Autodesk Fusion 360 part; units mm, degrees
(part 4 of 4)
  constraint coincident L729.end L734
  constraint perpendicular L729 L734
  constraint perpendicular L626 L768
  constraint coincident L630.end L658
  constraint perpendicular L630 L658
  constraint equal L626 L630
  constraint equal L626 L683
  constraint equal L626 L729
  constraint tangent L658 A42
  constraint tangent L690 A42
  constraint tangent A42 L768
  constraint coincident L694.end A42
  constraint coincident L694.start A42
  constraint coincident L622.end A42
  constraint coincident L622.start A42
  constraint tangent A42 L734
  constraint coincident P66 L622
  constraint coincident P66 L694
  constraint coincident P66 P37
  constraint vertical L701
  constraint perpendicular L648 L737
  constraint perpendicular L623 L718
  constraint perpendicular L623 L715
  constraint perpendicular L623 L672
  constraint perpendicular L648 L758
  constraint perpendicular L692 L737
  constraint equal L701 L718
  constraint equal L715 L718
  constraint equal L648 L718
  constraint symmetric L685.start L627.end L623
  constraint symmetric L672.start L627.start L623
  constraint symmetric L665.end L653.start L623
  constraint symmetric L665.start L653.end L623
  constraint symmetric L701.start L677.start L737
  constraint symmetric L677.end L673.start L737
  constraint symmetric L625.end L647.start L737
  constraint equal L672 L692
  constraint equal L692 L758
  constraint parallel L636 L648
  constraint equal L636 L692
  constraint symmetric L625.start L636.start L737
  constraint coincident L673.end L701
  constraint perpendicular L673 L701
  constraint coincident L644.end L718
  constraint coincident L676.end L715
  constraint perpendicular L676 L715
  constraint perpendicular L644 L718
  constraint coincident L650.end L648
  constraint perpendicular L648 L650
  constraint equal L644 L650
  constraint equal L644 L673
  constraint equal L644 L676
  constraint tangent L648 A43
  constraint tangent L701 A43
  constraint tangent L718 A43
  constraint coincident L737.end A43
  constraint coincident L737.start A43
  constraint coincident L623.end A43
  constraint coincident L623.start A43
  constraint tangent L715 A43
  constraint coincident P65 L623
  constraint coincident P65 L737
  constraint coincident P65 P38
  constraint vertical L649
  constraint perpendicular L643 L671
  constraint perpendicular L689 L691
  constraint perpendicular L678 L691
  constraint perpendicular L691 L725
  constraint perpendicular L643 L763
  constraint perpendicular L661 L671
  constraint equal L649 L689
  constraint equal L678 L689
  constraint equal L643 L689
  constraint symmetric L689.end L628.start L691
  constraint symmetric L640.start L628.end L691
  constraint symmetric L678.end L678.start L691
  constraint symmetric L698.start L704.end L691
  constraint symmetric L649.start L649.end L671
  constraint symmetric L661.start L645.start L671
  constraint symmetric L643.end L643.start L671
  constraint equal L661 L725
  constraint equal L661 L763
  constraint parallel L643 L724
  constraint equal L661 L724
  constraint symmetric L699.start L724.start L671
  constraint coincident L645.end L649
  constraint perpendicular L645 L649
  constraint coincident L640.end L689
  constraint coincident L705.end L678
  constraint perpendicular L678 L705
  constraint perpendicular L640 L689
  constraint coincident L720.end L643
  constraint perpendicular L643 L720
  constraint equal L640 L720
  constraint equal L640 L645
  constraint equal L640 L705
  constraint tangent A38 L643
  constraint tangent A38 L649
  constraint tangent A38 L689
  constraint coincident L671.end A38
  constraint coincident L671.start A38
  constraint coincident L691.end A38
  constraint coincident L691.start A38
  constraint tangent A38 L678
  constraint coincident P64 L691
  constraint coincident P64 L671
  constraint coincident P64 P39
  constraint vertical L660
  constraint perpendicular L687 L706
  constraint perpendicular L659 L756
  constraint perpendicular L659 L713
  constraint perpendicular L659 L761
  constraint perpendicular L651 L706
  constraint perpendicular L687 L711
  constraint equal L660 L756
  constraint equal L713 L756
  constraint equal L706 L756
  constraint symmetric L664.start L666.end L659
  constraint symmetric L664.end L632.start L659
  constraint symmetric L621.end L629.start L659
  constraint symmetric L621.start L629.end L659
  constraint symmetric L660.start L660.end L687
  constraint symmetric L711.start L668.start L687
  constraint symmetric L684.end L637.start L687
  constraint equal L711 L761
  constraint equal L651 L711
  constraint parallel L706 L714
  constraint equal L711 L714
  constraint symmetric L637.end L646.start L687
  constraint coincident L668.end L660
  constraint perpendicular L660 L668
  constraint coincident L632.end L756
  constraint coincident L669.end L713
  constraint perpendicular L669 L713
  constraint perpendicular L632 L756
  constraint coincident L646.end L706
  constraint perpendicular L646 L706
  constraint equal L632 L646
  constraint equal L632 L668
  constraint equal L632 L669
  constraint tangent A39 L706
  constraint tangent L660 A39
  constraint tangent A39 L756
  constraint coincident L687.end A39
  constraint coincident L687.start A39
  constraint coincident L659.end A39
  constraint coincident L659.start A39
  constraint tangent A39 L713
  constraint coincident P63 L659
  constraint coincident P63 L687
  constraint coincident P63 P36
  constraint vertical L693
  constraint perpendicular L657 L785
  constraint perpendicular L654 L777
  constraint perpendicular L654 L784
  constraint perpendicular L654 L782
  constraint perpendicular L657 L781
  constraint perpendicular L712 L785
  constraint equal L693 L777
  constraint equal L777 L784
  constraint equal L657 L777
  constraint symmetric L655.end L710.start L654
  constraint symmetric L710.end L655.start L654
  constraint symmetric L784.end L749.end L654
  constraint symmetric L781.start L736.start L654
  constraint symmetric L693.start L693.end L785
  constraint symmetric L712.end L712.start L785
  constraint symmetric L635.end L657.start L785
  constraint equal L712 L782
  constraint equal L712 L781
  constraint parallel L634 L657
  constraint equal L634 L712
  constraint symmetric L634.start L634.end L785
  constraint coincident L747.end L693
  constraint perpendicular L693 L747
  constraint coincident L792.end L777
  constraint coincident L736.end L784
  constraint perpendicular L736 L784
  constraint perpendicular L777 L792
  constraint coincident L776.end L657
  constraint perpendicular L657 L776
  constraint equal L776 L792
  constraint equal L747 L792
  constraint equal L736 L792
  constraint tangent L657 A45
  constraint tangent L693 A45
  constraint tangent L777 A45
  constraint coincident L785.end A45
  constraint coincident L785.start A45
  constraint coincident L654.end A45
  constraint coincident L654.start A45
  constraint tangent L784 A45
  constraint coincident P62 L654
  constraint coincident P62 L785
  constraint coincident P62 P40
  constraint vertical L778
  constraint perpendicular L641 L735
  constraint perpendicular L780 L787
  constraint perpendicular L787 L793
  constraint perpendicular L620 L787
  constraint perpendicular L641 L789
  constraint perpendicular L735 L783
  constraint equal L778 L780
  constraint equal L780 L793
  constraint equal L641 L780
  constraint symmetric L656.end L780.start L787
  constraint symmetric L620.start L620.end L787
  constraint symmetric L788.end L642.start L787
  constraint symmetric L775.start L642.end L787
  constraint symmetric L624.end L774.start L735
  constraint symmetric L624.start L774.end L735
  constraint symmetric L641.end L641.start L735
  constraint equal L620 L783
  constraint equal L783 L789
  constraint parallel L641 L779
  constraint equal L779 L783
  constraint symmetric L697.start L722.end L735
  constraint coincident L791.end L778
  constraint perpendicular L778 L791
  constraint coincident L795.end L780
  constraint coincident L775.end L793
  constraint perpendicular L775 L793
  constraint perpendicular L780 L795
  constraint coincident L731.end L641
  constraint perpendicular L641 L731
  constraint equal L731 L795
  constraint equal L791 L795
  constraint equal L775 L795
  constraint tangent L641 A44
  constraint tangent A44 L778
  constraint tangent A44 L780
  constraint coincident L735.end A44
  constraint coincident L735.start A44
  constraint coincident L787.end A44
  constraint coincident L787.start A44
  constraint tangent A44 L793
  constraint coincident P61 L787
  constraint coincident P61 L735
  constraint coincident P61 P41
  constraint vertical L723
  constraint perpendicular L638 L679
  constraint perpendicular L633 L695
  constraint perpendicular L633 L748
  constraint perpendicular L633 L702
  constraint perpendicular L638 L674
  constraint perpendicular L667 L679
  constraint equal L695 L723
  constraint equal L695 L748
  constraint equal L638 L695
  constraint symmetric L682.end L631.start L633
  constraint symmetric L662.start L631.end L633
  constraint symmetric L726.start L700.end L633
  constraint symmetric L674.end L674.start L633
  constraint symmetric L723.start L723.end L679
  constraint symmetric L667.start L667.end L679
  constraint symmetric L638.end L638.start L679
  constraint equal L667 L702
  constraint equal L667 L674
  constraint parallel L638 L738
  constraint equal L667 L738
  constraint symmetric L733.start L728.end L679
  constraint coincident L750.end L723
  constraint perpendicular L723 L750
  constraint coincident L662.end L695
  constraint coincident L686.end L748
  constraint perpendicular L686 L748
  constraint perpendicular L662 L695
  constraint coincident L757.end L638
  constraint perpendicular L638 L757
  constraint equal L662 L757
  constraint equal L662 L750
  constraint equal L662 L686
  constraint tangent L638 A40
  constraint tangent A40 L723
  constraint tangent L695 A40
  constraint coincident L679.end A40
  constraint coincident L679.start A40
  constraint coincident L633.end A40
  constraint coincident L633.start A40
  constraint tangent A40 L748
  constraint coincident P60 L633
  constraint coincident P60 L679
  constraint coincident P60 P42
  constraint vertical L760
  constraint perpendicular L764 L772
  constraint perpendicular L745 L770
  constraint perpendicular L770 L773
  constraint perpendicular L767 L770
  constraint perpendicular L766 L772
  constraint perpendicular L739 L764
  constraint equal L745 L760
  constraint equal L745 L773
  constraint equal L745 L772
  constraint symmetric L719.start L703.end L770
  constraint symmetric L719.end L703.start L770
  constraint symmetric L752.end L721.start L770
  constraint symmetric L721.end L752.start L770
  constraint symmetric L760.end L716.end L764
  constraint symmetric L739.start L716.start L764
  constraint symmetric L753.end L754.start L764
  constraint equal L739 L767
  constraint equal L739 L766
  constraint parallel L744 L772
  constraint equal L739 L744
  constraint symmetric L727.start L744.start L764
  constraint coincident L765.end L760
  constraint perpendicular L760 L765
  constraint coincident L742.end L745
  constraint coincident L769.end L773
  constraint perpendicular L769 L773
  constraint perpendicular L742 L745
  constraint coincident L727.end L772
  constraint perpendicular L727 L772
  constraint equal L727 L742
  constraint equal L742 L765
  constraint equal L742 L769
  constraint tangent A41 L772
  constraint tangent A41 L760
  constraint tangent A41 L745
  constraint coincident L764.end A41
  constraint coincident L764.start A41
  constraint coincident L770.end A41
  constraint coincident L770.start A41
  constraint tangent A41 L773
  constraint coincident P59 L770
  constraint coincident P59 L764
  constraint coincident P59 P43
  constraint vertical L811
  constraint perpendicular L818 L873
  constraint perpendicular L860 L879
  constraint perpendicular L834 L879
  constraint perpendicular L817 L879
  constraint perpendicular L854 L873
  constraint perpendicular L818 L832
  constraint equal L811 L860
  constraint equal L834 L860
  constraint equal L860 L873
  constraint symmetric L860.end L824.start L879
  constraint symmetric L817.end L817.start L879
  constraint symmetric L834.end L816.end L879
  constraint symmetric L796.start L854.start L879
  constraint symmetric L811.start L811.end L818
  constraint symmetric L812.end L821.start L818
  constraint symmetric L823.end L873.start L818
  constraint equal L817 L832
  constraint equal L832 L854
  constraint parallel L872 L873
  constraint equal L832 L872
  constraint symmetric L823.start L872.start L818
  constraint coincident L829.end L811
  constraint perpendicular L811 L829
  constraint coincident L870.end L860
  constraint coincident L796.end L834
  constraint perpendicular L796 L834
  constraint perpendicular L860 L870
  constraint coincident L867.end L873
  constraint perpendicular L867 L873
  constraint equal L867 L870
  constraint equal L829 L870
  constraint equal L796 L870
  constraint tangent A49 L873
  constraint tangent L811 A49
  constraint tangent A49 L860
  constraint coincident L818.end A49
  constraint coincident L818.start A49
  constraint coincident L879.end A49
  constraint coincident L879.start A49
  constraint tangent L834 A49
  constraint coincident P67 L879
  constraint coincident P67 L818
  constraint coincident P67 P46
  constraint vertical L826
  constraint perpendicular L842 L853
  constraint perpendicular L820 L825
  constraint perpendicular L825 L833
  constraint perpendicular L825 L845
  constraint perpendicular L806 L853
  constraint perpendicular L842 L863
  constraint equal L820 L826
  constraint equal L820 L833
  constraint equal L820 L853
  constraint symmetric L820.start L798.end L825
  constraint symmetric L845.start L798.start L825
  constraint symmetric L805.end L804.start L825
  constraint symmetric L804.end L805.start L825
  constraint symmetric L826.end L819.end L842
  constraint symmetric L835.end L797.start L842
  constraint symmetric L840.end L813.start L842
  constraint equal L845 L863
  constraint equal L806 L863
  constraint parallel L853 L866
  constraint equal L863 L866
  constraint symmetric L840.start L813.end L842
  constraint coincident L797.end L826
  constraint perpendicular L797 L826
  constraint coincident L852.end L820
  constraint coincident L814.end L833
  constraint perpendicular L814 L833
  constraint perpendicular L820 L852
  constraint coincident L846.end L853
  constraint perpendicular L846 L853
  constraint equal L846 L852
  constraint equal L797 L852
  constraint equal L814 L852
  constraint tangent A47 L853
  constraint tangent L826 A47
  constraint tangent L820 A47
  constraint coincident L842.end A47
  constraint coincident L842.start A47
  constraint coincident L825.end A47
  constraint coincident L825.start A47
  constraint tangent A47 L833
  constraint coincident P56 L825
  constraint coincident P56 L842
  constraint coincident P56 P47
  constraint vertical L800
  constraint perpendicular L822 L874
  constraint perpendicular L830 L881
  constraint perpendicular L828 L881
  constraint perpendicular L831 L881
  constraint perpendicular L827 L874
  constraint perpendicular L822 L848
  constraint equal L800 L830
  constraint equal L828 L830
  constraint equal L830 L874
  constraint symmetric L830.start L830.end L881
  constraint symmetric L831.end L831.start L881
  constraint symmetric L828.start L828.end L881
  constraint symmetric L827.start L807.start L881
  constraint symmetric L800.start L800.end L822
  constraint symmetric L847.end L848.end L822
  constraint symmetric L874.start L871.end L822
  constraint equal L831 L848
  constraint equal L827 L848
  constraint parallel L874 L880
  constraint equal L848 L880
  constraint symmetric L869.start L880.start L822
  constraint coincident L851.end L800
  constraint perpendicular L800 L851
  constraint coincident L883.end L830
  constraint coincident L807.end L828
  constraint perpendicular L807 L828
  constraint perpendicular L830 L883
  constraint coincident L869.end L874
  constraint perpendicular L869 L874
  constraint equal L869 L883
  constraint equal L851 L883
  constraint equal L807 L883
  constraint tangent A46 L874
  constraint tangent L800 A46
  constraint tangent A46 L830
  constraint coincident L822.end A46
  constraint coincident L822.start A46
  constraint coincident L881.end A46
  constraint coincident L881.start A46
  constraint tangent A46 L828
  constraint coincident P58 L881
  constraint coincident P58 L822
  constraint coincident P58 P44
  constraint vertical L858
  constraint perpendicular L810 L843
  constraint perpendicular L802 L809
  constraint perpendicular L809 L839
  constraint perpendicular L799 L809
  constraint perpendicular L810 L864
  constraint perpendicular L808 L843
  constraint equal L802 L858
  constraint equal L802 L839
  constraint equal L802 L810
  constraint symmetric L802.end L802.start L809
  constraint symmetric L799.start L799.end L809
  constraint symmetric L839.start L839.end L809
  constraint symmetric L855.start L857.end L809
  constraint symmetric L803.start L850.end L843
  constraint symmetric L808.end L803.end L843
  constraint symmetric L810.end L801.start L843
  constraint equal L799 L808
  constraint equal L808 L864
  constraint parallel L810 L836
  constraint equal L808 L836
  constraint symmetric L801.end L815.start L843
  constraint coincident L841.end L858
  constraint perpendicular L841 L858
  constraint coincident L838.end L802
  constraint coincident L861.end L839
  constraint perpendicular L839 L861
  constraint perpendicular L802 L838
  constraint coincident L849.end L810
  constraint perpendicular L810 L849
  constraint equal L838 L849
  constraint equal L838 L841
  constraint equal L838 L861
  constraint tangent L810 A48
  constraint tangent A48 L858
  constraint tangent L802 A48
  constraint coincident L843.end A48
  constraint coincident L843.start A48
  constraint coincident L809.end A48
  constraint coincident L809.start A48
  constraint tangent A48 L839
  constraint coincident P57 L809
  constraint coincident P57 L843
  constraint coincident P57 P45
  constraint equal A42 A50
  constraint equal A43 A51
  constraint equal A38 A52
  constraint equal A39 A53
  constraint equal A45 A54
  constraint equal A44 A55
  constraint equal A40 A56
  constraint equal A41 A57
  constraint equal A46 A58
  constraint equal A48 A59
  constraint equal A47 A60
  constraint equal A49 A61
  constraint equal A37 A62
  constraint equal A34 A63
  constraint equal A35 A64
  constraint equal A36 A65
  constraint equal A33 A66
  constraint equal A32 A67
  constraint equal A31 A68
  constraint equal A30 A69
  measures "d105" distance of L8.start L8.end
  measures "d106" distance of L10.end L11.end
  measures "d371" distance of L11.end L23.end
  measures "d372" distance of L37.start L36.end
  measures "d373" distance of L37.end L32.start
  measures "d374" distance of L32.end L32.start
  measures "d375" distance of L51.start L48.end
  measures "d376" distance of L48.start L51.end
  measures "d377" distance of L48.start L63.end
  measures "d378" distance of L73.start L70.end
  measures "d379" distance of L70.start L73.end
  measures "d380" distance of L70.start L85.end
  measures "d381" distance of L95.start L92.end
  measures "d382" distance of L92.start L95.end
  measures "d383" distance of L92.start L107.end
  measures "d384" distance of L117.start L114.end
  measures "d385" distance of L114.start L117.end
  measures "d386" distance of L114.start L129.end
  measures "d387" distance of L139.start L136.end
  measures "d388" distance of L136.start L139.end
  measures "d389" distance of L136.start L151.end
  measures "d390" distance of L161.start L158.end
  measures "d391" distance of L158.start L161.end
  measures "d392" distance of L158.start L173.end
  measures "d393" distance of L183.start L180.end
  measures "d394" distance of L180.start L183.end
  measures "d395" distance of L180.start L195.end
  measures "d396" distance of L205.start L202.end
  measures "d397" distance of L202.start L205.end
  measures "d398" distance of L202.start L217.end
  measures "d504" distance of L224.start L235.end
  measures "d505" distance of L230.start L224.end
  measures "d506" distance of L230.start L230.end
  measures "d507" distance of L246.start L257.end
  measures "d508" distance of L252.start L246.end
  measures "d509" distance of L252.start L252.end
  measures "d510" distance of L268.start L279.end
  measures "d511" distance of L274.start L268.end
  measures "d512" distance of L274.start L274.end
  measures "d513" distance of L290.start L301.end
  measures "d514" distance of L296.start L290.end
  measures "d515" distance of L296.start L296.end
  measures "d516" distance of L312.start L323.end
  measures "d517" distance of L318.start L312.end
  measures "d518" distance of L318.start L318.end
  measures "d519" distance of L334.start L345.end
  measures "d520" distance of L340.start L334.end
  measures "d521" distance of L340.start L340.end
  measures "d522" distance of L356.start L367.end
  measures "d523" distance of L362.start L356.end
  measures "d524" distance of L362.start L362.end
  measures "d525" distance of L378.start L389.end
  measures "d526" distance of L384.start L378.end
  measures "d527" distance of L384.start L384.end
  measures "d528" distance of L400.start L411.end
  measures "d529" distance of L406.start L400.end
  measures "d530" distance of L406.start L406.end
  measures "d531" distance of L422.start L433.end
  measures "d532" distance of L428.start L422.end
  measures "d533" distance of L428.start L428.end
  measures "d568" distance of L450.end L452.start
  measures "d569" distance of L450.start L459.end
  measures "d570" distance of L450.start L457.end
  measures "d571" distance of L477.end L481.start
  measures "d572" distance of L477.start L482.start
  measures "d573" distance of L477.start L478.end
  measures "d574" distance of L495.end L499.start
  measures "d575" distance of L495.start L510.start
  measures "d576" distance of L495.start L528.end
  measures "d577" distance of L513.start L513.end
  measures "d578" distance of L496.start L496.end
  measures "d579" distance of L496.end L523.end
  measures "d580" distance of L542.end L581.start
  measures "d581" distance of L542.start L588.start
  measures "d582" distance of L542.start L561.end
  measures "d583" distance of L576.start L539.end
  measures "d584" distance of L601.end L539.start
  measures "d585" distance of L539.start L540.end
  measures "d586" distance of L549.end L549.start
  measures "d587" distance of L555.start L562.start
  measures "d588" distance of L555.start L555.end
  measures "d589" distance of L591.start L586.end
  measures "d590" distance of L589.start L586.start
  measures "d591" distance of L615.end L586.start
  measures "d592" distance of L652.end L663.start
  measures "d593" distance of L626.start L663.end
  measures "d594" distance of L626.start L626.end
  measures "d595" distance of L685.start L627.end
  measures "d596" distance of L672.start L627.start
  measures "d597" distance of L627.start L644.end
  measures "d598" distance of L689.end L628.start
  measures "d599" distance of L640.start L628.end
  measures "d600" distance of L640.start L640.end
  measures "d601" distance of L664.start L666.end
  measures "d602" distance of L664.end L632.start
  measures "d603" distance of L632.end L632.start
  measures "d604" distance of L655.end L710.start
  measures "d605" distance of L710.end L655.start
  measures "d606" distance of L792.end L655.start
  measures "d607" distance of L656.end L780.start
  measures "d608" distance of L620.start L620.end
  measures "d609" distance of L620.end L795.end
  measures "d610" distance of L682.end L631.start
  measures "d611" distance of L662.start L631.end
  measures "d612" distance of L662.start L662.end
  measures "d613" distance of L719.start L703.end
  measures "d614" distance of L719.end L703.start
  measures "d615" distance of L742.end L703.start
  measures "d616" distance of L860.end L824.start
  measures "d617" distance of L817.end L817.start
  measures "d618" distance of L817.end L870.end
  measures "d619" distance of L820.start L798.end
  measures "d620" distance of L845.start L798.start
  measures "d621" distance of L852.end L798.start
  measures "d622" distance of L830.start L830.end
  measures "d623" distance of L831.end L831.start
  measures "d624" distance of L831.end L883.end
  measures "d625" distance of L802.end L802.start
  measures "d626" distance of L799.start L799.end
  measures "d627" distance of L799.end L838.end
extrude "돌출4" add sketch "스케치1" along normal blind 0.4 contours L0 L1 L2 L3 | L40 L41 L42 L43
extrude "돌출7" add sketch "스케치1" along normal blind 0.4 and the other way blind 0 contours A42 | A43
extrude "돌출6" cut sketch "스케치2" along normal through all contours A40 | L0 L3 L160 | L0 L3 A0 L160 | L0 L1 A0 | A0 | L2 L3 A0 | L1 L2 A0 | A44 | L4 L7 L174 | L4 L7 A1 L174 | L4 L5 A1 | A1 | L6 L7 A1 | L5 L6 A1 | A45 | L8 L11 L175 | L8 L11 A2 L175 | L8 L9 A2 | A2 | L10 L11 A2 | L9 L10 A2 | A46 | L12 L15 L176 | L12 L15 A3 L176 | L12 L13 A3 | A3 | L14 L15 A3 | L13 L14 A3 | A47 | L16 L19 L177 | L16 L19 A4 L177 | L16 L17 A4 | A4 | L18 L19 A4 | L17 L18 A4 | A48 | L20 L23 L178 | L20 L23 A5 L178 | L20 L21 A5 | A5 | L22 L23 A5 | L21 L22 A5 | A49 | L24 L27 L179 | L24 L27 A6 L179 | L24 L25 A6 | A6 | L26 L27 A6 | L25 L26 A6 | A50 | L28 L31 L180 | L28 L31 A7 L180 | L28 L29 A7 | A7 | L30 L31 A7 | L29 L30 A7 | A51 | L32 L35 L181 | L32 L35 A8 L181 | L32 L33 A8 | A8 | L34 L35 A8 | L33 L34 A8 | A52 | L36 L39 L182 | L36 L39 A9 L182 | L36 L37 A9 | A9 | L38 L39 A9 | L37 L38 A9 | A53 | L40 L43 L192 | L40 L43 A10 L192 | L40 L41 A10 | A10 | L42 L43 A10 | L41 L42 A10 | A54 | L44 L47 L169 | L44 L47 A11 L169 | L44 L45 A11 | A11 | L46 L47 A11 | L45 L46 A11 | A55 | L48 L51 L193 | L48 L51 A12 L193 | L48 L49 A12 | A12 | L50 L51 A12 | L49 L50 A12 | A56 | L52 L55 L170 | L52 L55 A13 L170 | L52 L53 A13 | A13 | L54 L55 A13 | L53 L54 A13 | A57 | L56 L59 L194 | L56 L59 A14 L194 | L56 L57 A14 | A14 | L58 L59 A14 | L57 L58 A14 | A58 | L60 L63 L171 | L60 L63 A15 L171 | L60 L61 A15 | A15 | L62 L63 A15 | L61 L62 A15 | A59 | L64 L67 L195 | L64 L67 A16 L195 | L64 L65 A16 | A16 | L66 L67 A16 | L65 L66 A16 | A60 | L68 L71 L172 | L68 L71 A17 L172 | L68 L69 A17 | A17 | L70 L71 A17 | L69 L70 A17 | A61 | L72 L75 L196 | L72 L75 A18 L196 | L72 L73 A18 | A18 | L74 L75 A18 | L73 L74 A18 | A42 | L76 L79 L162 | L76 L79 A19 L162 | L76 L77 A19 | A19 | L78 L79 A19 | L77 L78 A19 | A69 | L80 L83 L213 | L80 L83 A29 L213 | L80 L81 A29 | A29 | L82 L83 A29 | L81 L82 A29 | A70 | L84 L87 L212 | L84 L87 A28 L212 | L84 L85 A28 | A28 | L86 L87 A28 | L85 L86 A28 | A67 | L88 L91 L211 | L88 L91 A27 L211 | L88 L89 A27 | A27 | L90 L91 A27 | L89 L90 A27 | A68 | L92 L95 L210 | L92 L95 A26 L210 | L92 L93 A26 | A26 | L94 L95 A26 | L93 L94 A26 | A65 | L96 L99 L209 | L96 L99 A25 L209 | L96 L97 A25 | A25 | L98 L99 A25 | L97 L98 A25 | A66 | L100 L103 L208 | L100 L103 A23 L208 | L100 L101 A23 | A23 | L102 L103 A23 | L101 L102 A23 | A63 | L104 L107 L207 | L104 L107 A24 L207 | L104 L105 A24 | A24 | L106 L107 A24 | L105 L106 A24 | A64 | L108 L111 L173 | L108 L111 A22 L173 | L108 L109 A22 | A22 | L110 L111 A22 | L109 L110 A22 | A62 | L112 L115 L206 | L112 L115 A21 L206 | L112 L113 A21 | A21 | L114 L115 A21 | L113 L114 A21 | A41 | L116 L119 L165 | L116 L119 A20 L165 | L116 L117 A20 | A20 | L118 L119 A20 | L117 L118 A20 | A79 | L120 L123 L231 | L120 L123 A30 L231 | L120 L121 A30 | A30 | L122 L123 A30 | L121 L122 A30 | A78 | L124 L127 L230 | L124 L127 A31 L230 | L124 L125 A31 | A31 | L126 L127 A31 | L125 L126 A31 | A77 | L128 L131 L229 | L128 L131 A32 L229 | L128 L129 A32 | A32 | L130 L131 A32 | L129 L130 A32 | A76 | L132 L135 L228 | L132 L135 A33 L228 | L132 L133 A33 | A33 | L134 L135 A33 | L133 L134 A33 | A75 | L136 L139 L227 | L136 L139 A34 L227 | L136 L137 A34 | A34 | L138 L139 A34 | L137 L138 A34 | A74 | L140 L143 L226 | L140 L143 A35 L226 | L140 L141 A35 | A35 | L142 L143 A35 | L141 L142 A35 | A73 | L144 L147 L225 | L144 L147 A36 L225 | L144 L145 A36 | A36 | L146 L147 A36 | L145 L146 A36 | A72 | L148 L151 L224 | L148 L151 A37 L224 | L148 L149 A37 | A37 | L150 L151 A37 | L149 L150 A37 | A71 | L152 L155 L223 | L152 L155 A38 L223 | L152 L153 A38 | A38 | L154 L155 A38 | L153 L154 A38 | A43 | L156 L159 L167 | L156 L159 A39 L167 | L156 L157 A39 | A39 | L158 L159 A39 | L157 L158 A39
extrude "돌출8" add sketch "스케치2" along normal blind 0.4 contours A40 | L0 L3 L160 | A44 | L4 L7 L174 | A45 | L8 L11 L175 | A46 | L12 L15 L176 | A47 | L16 L19 L177 | A48 | L20 L23 L178 | A49 | L24 L27 L179 | A50 | L28 L31 L180 | A51 | L32 L35 L181 | A52 | L36 L39 L182 | A53 | L40 L43 L192 | A54 | L44 L47 L169 | A55 | L48 L51 L193 | A56 | L52 L55 L170 | A57 | L56 L59 L194 | A58 | L60 L63 L171 | A59 | L64 L67 L195 | A60 | L68 L71 L172 | A61 | L72 L75 L196 | A42 | L76 L79 L162 | A69 | L80 L83 L213 | A70 | L84 L87 L212 | A67 | L88 L91 L211 | A68 | L92 L95 L210 | A65 | L96 L99 L209 | A66 | L100 L103 L208 | A63 | L104 L107 L207 | A64 | L108 L111 L173 | A62 | L112 L115 L206 | A41 | L116 L119 L165 | A79 | L120 L123 L231 | A78 | L124 L127 L230 | A77 | L128 L131 L229 | A76 | L132 L135 L228 | A75 | L136 L139 L227 | A74 | L140 L143 L226 | A73 | L144 L147 L225 | A72 | L148 L151 L224 | A71 | L152 L155 L223 | A43 | L156 L159 L167
extrude "돌출9" add sketch "스케치2" against normal blind 2 contours A40 | A44 | A45 | A46 | A47 | A48 | A49 | A50 | A51 | A52 | A53 | A54 | A55 | A56 | A57 | A58 | A59 | A60 | A61 | A42 | A69 | A70 | A67 | A68 | A65 | A66 | A63 | A64 | A62 | A41 | A79 | A78 | A77 | A76 | A75 | A74 | A73 | A72 | A71 | A43
extrude "돌출11" add sketch "스케치3" along normal blind 0.4 contours L0 L10 L11 L12 | L3 L16 L17 L18 | L1 L19 L20 L21 | L2 L13 L14 L15 | L26 L27 L31 L45 | L28 L34 L40 L44 | L30 L33 L35 L39 | L36 L37 L43 L47 | L48 L51 L52 L56 | L50 L54 L57 L58 | L55 L59 L60 L61 | L66 L67 L68 L69 | L70 L73 L74 L78 | L72 L76 L79 L80 | L77 L81 L82 L83 | L88 L89 L90 L91 | L92 L95 L96 L100 | L94 L98 L101 L102 | L99 L103 L104 L105 | L110 L111 L112 L113 | L114 L117 L118 L122 | L116 L120 L123 L124 | L121 L125 L126 L127 | L132 L133 L134 L135 | L136 L139 L140 L144 | L138 L142 L145 L146 | L143 L147 L148 L149 | L154 L155 L156 L157 | L158 L161 L162 L166 | L160 L164 L167 L168 | L165 L169 L170 L171 | L176 L177 L178 L179 | L180 L183 L184 L188 | L182 L186 L189 L190 | L187 L191 L192 L193 | L198 L199 L200 L201 | L202 L205 L206 L210 | L204 L208 L211 L212 | L209 L213 L214 L215 | L220 L221 L222 L223 | L224 L235 A21 | L224 L242 L243 A21 | L235 L242 A21 | L227 L244 A21 | L229 L231 L244 A21 | L227 L231 A21 | L226 L239 L240 A21 | L234 L240 A21 | L234 L239 A21 | L237 L241 A21 | L228 L232 L237 A21 | L232 L241 A21 | L246 L257 A22 | L246 L264 L265 A22 | L257 L264 A22 | L249 L266 A22 | L251 L253 L266 A22 | L249 L253 A22 | L248 L261 L262 A22 | L256 L262 A22 | L256 L261 A22 | L259 L263 A22 | L250 L254 L259 A22 | L254 L263 A22 | L268 L279 A23 | L268 L286 L287 A23 | L279 L286 A23 | L271 L288 A23 | L273 L275 L288 A23 | L271 L275 A23 | L270 L283 L284 A23 | L278 L284 A23 | L278 L283 A23 | L281 L285 A23 | L272 L276 L281 A23 | L276 L285 A23 | L290 L301 A24 | L290 L308 L309 A24 | L301 L308 A24 | L293 L310 A24 | L295 L297 L310 A24 | L293 L297 A24 | L292 L305 L306 A24 | L300 L306 A24 | L300 L305 A24 | L303 L307 A24 | L294 L298 L303 A24 | L298 L307 A24 | L312 L323 A20 | L312 L330 L331 A20 | L323 L330 A20 | L315 L332 A20 | L317 L319 L332 A20 | L315 L319 A20 | L314 L327 L328 A20 | L322 L328 A20 | L322 L327 A20 | L325 L329 A20 | L316 L320 L325 A20 | L320 L329 A20 | L334 L345 A25 | L334 L352 L353 A25 | L345 L352 A25 | L337 L354 A25 | L339 L341 L354 A25 | L337 L341 A25 | L336 L349 L350 A25 | L344 L350 A25 | L344 L349 A25 | L347 L351 A25 | L338 L342 L347 A25 | L342 L351 A25 | L356 L367 A26 | L356 L374 L375 A26 | L367 L374 A26 | L359 L376 A26 | L361 L363 L376 A26 | L359 L363 A26 | L358 L371 L372 A26 | L366 L372 A26 | L366 L371 A26 | L369 L373 A26 | L360 L364 L369 A26 | L364 L373 A26 | L378 L389 A27 | L378 L396 L397 A27 | L389 L396 A27 | L381 L398 A27 | L383 L385 L398 A27 | L381 L385 A27 | L380 L393 L394 A27 | L388 L394 A27 | L388 L393 A27 | L391 L395 A27 | L382 L386 L391 A27 | L386 L395 A27 | L400 L411 A28 | L400 L418 L419 A28 | L411 L418 A28 | L403 L420 A28 | L405 L407 L420 A28 | L403 L407 A28 | L402 L415 L416 A28 | L410 L416 A28 | L410 L415 A28 | L413 L417 A28 | L404 L408 L413 A28 | L408 L417 A28 | L422 L433 A29 | L422 L440 L441 A29 | L433 L440 A29 | L425 L442 A29 | L427 L429 L442 A29 | L425 L429 A29 | L424 L437 L438 A29 | L432 L438 A29 | L432 L437 A29 | L435 L439 A29 | L426 L430 L435 A29 | L430 L439 A29 | L444 L447 L456 A69 | L444 L453 A69 | L460 L461 L465 A69 | L461 L464 A69 | L447 L453 A69 | L460 L464 A69 | L448 L455 A69 | L449 L451 L455 A69 | L448 L449 A69 | L450 L459 L462 A69 | L452 L459 A69 | L450 L452 A69 | L466 L476 L480 A68 | L466 L470 A68 | L469 L475 L486 A68 | L469 L474 A68 | L470 L476 A68 | L474 L486 A68 | L471 L472 A68 | L471 L473 L487 A68 | L472 L473 A68 | L477 L482 L484 A68 | L481 L484 A68 | L477 L481 A68 | L488 L491 A67 | L491 L493 L529 A67 | L488 L529 A67 | L495 L499 A67 | L495 L510 L518 A67 | L497 L503 L512 A67 | L492 L497 A67 | L499 L518 A67 | L492 L512 A67 | L506 L522 A67 | L505 L506 L508 A67 | L508 L522 A67 | L494 L507 L515 A66 | L494 L501 A66 | L500 L502 L509 A66 | L509 L517 A66 | L501 L515 A66 | L500 L517 A66 | L511 L524 A66 | L511 L516 L525 A66 | L516 L524 A66 | L496 L527 L531 A66 | L513 L527 A66 | L513 L531 A66 | L532 L614 A64 | L570 L587 L614 A64 | L532 L587 A64 | L539 L576 A64 | L539 L601 L609 A64 | L547 L550 L566 A64 | L550 L571 A64 | L576 L601 A64 | L547 L571 A64 | L538 L602 A64 | L538 L556 L567 A64 | L556 L602 A64 | L533 L545 L560 A65 | L533 L535 A65 | L548 L594 L604 A65 | L548 L554 A65 | L535 L545 A65 | L554 L604 A65 | L542 L581 A65 | L542 L588 L592 A65 | L581 L592 A65 | L569 L575 L598 A65 | L574 L575 A65 | L569 L574 A65 | L537 L590 A63 | L537 L544 L563 A63 | L563 L590 A63 | L546 L595 A63 | L568 L585 L595 A63 | L546 L568 A63 | L541 L543 L579 A63 | L543 L564 A63 | L541 L564 A63 | L549 L603 A63 | L562 L596 L603 A63 | L549 L596 A63 | L565 L584 L619 A62 | L565 L616 A62 | L586 L589 L591 A62 | L591 L611 A62 | L584 L616 A62 | L586 L611 A62 | L610 L617 A62 | L608 L613 L617 A62 | L610 L613 A62 | L577 L593 L606 A62 | L577 L605 A62 | L605 L606 A62 | L620 L656 L794 A55 | L780 L794 A55 | L656 L780 A55 | L624 L778 A55 | L624 L774 L783 A55 | L697 L722 L779 A55 | L641 L722 A55 | L774 L778 A55 | L641 L697 A55 | L788 L793 A55 | L642 L788 L789 A55 | L642 L793 A55 | L621 L629 L651 A53 | L621 L713 A53 | L680 L711 L743 A53 | L660 L743 A53 | L629 L713 A53 | L660 L680 A53 | L684 L706 A53 | L637 L684 L714 A53 | L637 L706 A53 | L664 L666 L761 A53 | L664 L756 A53 | L666 L756 A53 | L625 L636 L647 A51 | L625 L648 A51 | L653 L665 L758 A51 | L653 L715 A51 | L647 L648 A51 | L665 L715 A51 | L627 L718 A51 | L627 L672 L685 A51 | L685 L718 A51 | L677 L692 L707 A51 | L677 L701 A51 | L701 L707 A51 | L628 L689 A52 | L628 L725 L741 A52 | L689 L741 A52 | L649 L746 A52 | L661 L670 L746 A52 | L649 L670 A52 | L699 L724 L751 A52 | L643 L751 A52 | L643 L699 A52 | L678 L698 A52 | L698 L704 L763 A52 | L678 L704 A52 | L631 L695 A56 | L631 L682 L702 A56 | L682 L695 A56 | L723 L755 A56 | L667 L740 L755 A56 | L723 L740 A56 | L728 L733 L738 A56 | L638 L728 A56 | L638 L733 A56 | L700 L748 A56 | L674 L700 L726 A56 | L726 L748 A56 | L634 L635 L790 A54 | L657 L790 A54 | L635 L657 A54 | L655 L777 A54 | L655 L710 L782 A54 | L749 L781 L786 A54 | L784 L786 A54 | L710 L777 A54 | L749 L784 A54 | L693 L759 A54 | L712 L730 L759 A54 | L693 L730 A54 | L639 L675 L681 A50 | L639 L658 A50 | L688 L696 L708 A50 | L708 L734 A50 | L658 L675 A50 | L688 L734 A50 | L652 L768 A50 | L652 L663 L732 A50 | L663 L768 A50 | L709 L717 L762 A50 | L690 L762 A50 | L690 L717 A50 | L703 L719 L767 A57 | L703 L745 A57 | L744 L753 L754 A57 | L754 L772 A57 | L719 L745 A57 | L753 L772 A57 | L716 L760 A57 | L716 L739 L771 A57 | L760 L771 A57 | L721 L752 L766 A57 | L721 L773 A57 | L752 L773 A57 | L798 L845 L862 A60 | L798 L820 A60 | L813 L840 L866 A60 | L813 L853 A60 | L820 L862 A60 | L840 L853 A60 | L819 L826 A60 | L819 L835 L863 A60 | L826 L835 A60 | L804 L805 L806 A60 | L804 L833 A60 | L805 L833 A60 | L799 L837 L859 A59 | L802 L837 A59 | L802 L859 A59 | L850 L858 A59 | L803 L808 L850 A59 | L801 L815 L836 A59 | L801 L810 A59 | L803 L858 A59 | L810 L815 A59 | L839 L855 A59 | L855 L857 L864 A59 | L839 L857 A59 | L800 L856 A58 | L800 L847 A58 | L847 L848 L856 A58 | L831 L844 L878 A58 | L830 L844 A58 | L828 L865 A58 | L827 L865 L875 A58 | L830 L878 A58 | L828 L875 A58 | L871 L880 L882 A58 | L874 L882 A58 | L871 L874 A58 | L811 L821 A61 | L811 L812 A61 | L812 L821 L832 A61 | L817 L824 L868 A61 | L824 L860 A61 | L816 L834 A61 | L816 L854 L877 A61 | L860 L868 A61 | L834 L877 A61 | L823 L872 L876 A61 | L873 L876 A61 | L823 L873 A61
move_body "이동1" bodies 1 to x (1, 0, 0) y (0, -1, 0) z (0, 0, -1) at (0, 138, 0.8)
move_body "이동2" bodies 1 to x (1, 0, 0) y (0, 1, 0) z (0, 0, 1) at (0, -69, -0.4)
equation "d6 = RADIUS"
equation "d38 = HEIGHT"
equation "d46 = HEIGHT"
equation "d51 = DEGR"
equation "d55 = DEGR"
equation "d57 = HEIGHT"
equation "d59 = -( COL + 1 mm )"
equation "RADIUS = 10.1 mm"
equation "d63 = DEGR"
equation "d64 = DEGR"
equation "d65 = DEGR"
equation "d66 = DEGR"
equation "d67 = DEGR"
equation "d68 = DEGR"
equation "d69 = DEGR"
equation "d70 = DEGR"
equation "d72 = DEGR"
equation "DEGR = 45 deg"
equation "d74 = DEGR"
equation "d75 = DEGR"
equation "d76 = DEGR"
equation "d77 = DEGR"
equation "d78 = DEGR"
equation "d80 = DEGR"
equation "d81 = DEGR"
equation "d82 = DEGR"
equation "d83 = DEGR"
equation "d84 = DEGR"
equation "d85 = DEGR"
equation "d86 = DEGR"
equation "d87 = DEGR"
equation "d88 = DEGR"
equation "d89 = DEGR"
equation "d91 = DEGR"
equation "d92 = DEGR"
equation "d93 = DEGR"
equation "d94 = DEGR"
equation "d95 = DEGR"
equation "d96 = DEGR"
equation "d97 = DEGR"
equation "d98 = DEGR"
equation "d99 = DEGR"
equation "d100 = DEGR"
equation "d101 = DEGR"
equation "d102 = DEGR"
equation "HEIGHT = 0.4 mm"
equation "COL = 1.0 mm"
equation "d105 = SLOT_WIDTH_UPPER"
equation "d106 = SLOT_WIDTH_LOWER"
equation "SLOT_WIDTH_UPPER = 2.7 mm"
equation "SLOT_WIDTH_LOWER = 2 mm"
equation "d371 = SLOT_SIZE"
equation "d372 = SLOT_WIDTH_UPPER"
equation "d373 = SLOT_WIDTH_LOWER"
equation "d374 = SLOT_SIZE"
equation "d375 = SLOT_WIDTH_UPPER"
equation "d376 = SLOT_WIDTH_LOWER"
equation "d377 = SLOT_SIZE"
equation "d378 = SLOT_WIDTH_UPPER"
equation "d379 = SLOT_WIDTH_LOWER"
equation "d380 = SLOT_SIZE"
equation "d381 = SLOT_WIDTH_UPPER"
equation "d382 = SLOT_WIDTH_LOWER"
equation "d383 = SLOT_SIZE"
equation "d384 = SLOT_WIDTH_UPPER"
equation "d385 = SLOT_WIDTH_LOWER"
equation "d386 = SLOT_SIZE"
equation "d387 = SLOT_WIDTH_UPPER"
equation "d388 = SLOT_WIDTH_LOWER"
equation "d389 = SLOT_SIZE"
equation "d390 = SLOT_WIDTH_UPPER"
equation "d391 = SLOT_WIDTH_LOWER"
equation "d392 = SLOT_SIZE"
equation "d393 = SLOT_WIDTH_UPPER"
equation "d394 = SLOT_WIDTH_LOWER"
equation "d395 = SLOT_SIZE"
equation "d396 = SLOT_WIDTH_UPPER"
equation "d397 = SLOT_WIDTH_LOWER"
equation "d398 = SLOT_SIZE"
equation "d504 = SLOT_WIDTH_UPPER"
equation "d505 = SLOT_WIDTH_LOWER"
equation "d506 = SLOT_SIZE"
equation "d507 = SLOT_WIDTH_UPPER"
equation "d508 = SLOT_WIDTH_LOWER"
equation "d509 = SLOT_SIZE"
equation "d510 = SLOT_WIDTH_UPPER"
equation "d511 = SLOT_WIDTH_LOWER"
equation "d512 = SLOT_SIZE"
equation "d513 = SLOT_WIDTH_UPPER"
equation "d514 = SLOT_WIDTH_LOWER"
equation "d515 = SLOT_SIZE"
equation "d516 = SLOT_WIDTH_UPPER"
equation "d517 = SLOT_WIDTH_LOWER"
equation "d518 = SLOT_SIZE"
equation "d519 = SLOT_WIDTH_UPPER"
equation "d520 = SLOT_WIDTH_LOWER"
equation "d521 = SLOT_SIZE"
equation "d522 = SLOT_WIDTH_UPPER"
equation "d523 = SLOT_WIDTH_LOWER"
equation "d524 = SLOT_SIZE"
equation "d525 = SLOT_WIDTH_UPPER"
equation "d526 = SLOT_WIDTH_LOWER"
equation "d527 = SLOT_SIZE"
equation "d528 = SLOT_WIDTH_UPPER"
equation "d529 = SLOT_WIDTH_LOWER"
equation "d530 = SLOT_SIZE"
equation "d531 = SLOT_WIDTH_UPPER"
equation "d532 = SLOT_WIDTH_LOWER"
equation "d533 = SLOT_SIZE"
equation "d568 = SLOT_WIDTH_UPPER"
equation "d569 = SLOT_WIDTH_LOWER"
equation "d570 = SLOT_SIZE"
equation "d571 = SLOT_WIDTH_UPPER"
equation "d572 = SLOT_WIDTH_LOWER"
equation "d573 = SLOT_SIZE"
equation "d574 = SLOT_WIDTH_UPPER"
equation "d575 = SLOT_WIDTH_LOWER"
equation "d576 = SLOT_SIZE"
equation "d577 = SLOT_WIDTH_UPPER"
equation "d578 = SLOT_WIDTH_LOWER"
equation "d579 = SLOT_SIZE"
equation "d580 = SLOT_WIDTH_UPPER"
equation "d581 = SLOT_WIDTH_LOWER"
equation "d582 = SLOT_SIZE"
equation "d583 = SLOT_WIDTH_UPPER"
equation "d584 = SLOT_WIDTH_LOWER"
equation "d585 = SLOT_SIZE"
equation "d586 = SLOT_WIDTH_UPPER"
equation "d587 = SLOT_WIDTH_LOWER"
equation "d588 = SLOT_SIZE"
equation "d589 = SLOT_WIDTH_UPPER"
equation "d590 = SLOT_WIDTH_LOWER"
equation "d591 = SLOT_SIZE"
equation "d592 = SLOT_WIDTH_UPPER"
equation "d593 = SLOT_WIDTH_LOWER"
equation "d594 = SLOT_SIZE"
equation "d595 = SLOT_WIDTH_UPPER"
equation "d596 = SLOT_WIDTH_LOWER"
equation "d597 = SLOT_SIZE"
equation "d598 = SLOT_WIDTH_UPPER"
equation "d599 = SLOT_WIDTH_LOWER"
equation "d600 = SLOT_SIZE"
equation "d601 = SLOT_WIDTH_UPPER"
equation "d602 = SLOT_WIDTH_LOWER"
equation "d603 = SLOT_SIZE"
equation "d604 = SLOT_WIDTH_UPPER"
equation "d605 = SLOT_WIDTH_LOWER"
equation "d606 = SLOT_SIZE"
equation "d607 = SLOT_WIDTH_UPPER"
equation "d608 = SLOT_WIDTH_LOWER"
equation "d609 = SLOT_SIZE"
equation "d610 = SLOT_WIDTH_UPPER"
equation "d611 = SLOT_WIDTH_LOWER"
equation "d612 = SLOT_SIZE"
equation "d613 = SLOT_WIDTH_UPPER"
equation "d614 = SLOT_WIDTH_LOWER"
equation "d615 = SLOT_SIZE"
equation "d616 = SLOT_WIDTH_UPPER"
equation "d617 = SLOT_WIDTH_LOWER"
equation "d618 = SLOT_SIZE"
equation "d619 = SLOT_WIDTH_UPPER"
equation "d620 = SLOT_WIDTH_LOWER"
equation "d621 = SLOT_SIZE"
equation "d622 = SLOT_WIDTH_UPPER"
equation "d623 = SLOT_WIDTH_LOWER"
equation "d624 = SLOT_SIZE"
equation "d625 = SLOT_WIDTH_UPPER"
equation "d626 = SLOT_WIDTH_LOWER"
equation "d627 = SLOT_SIZE"
equation "d628 = HEIGHT"
equation "SLOT_SIZE = 1.05 mm"
named bodies: "Seat"
